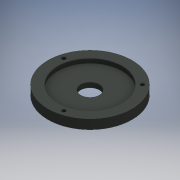
# Autodesk Inventor part: fix_plate
Saved by Autodesk Inventor 2018 (Build 220112000, 112)
## iProperties
Created: 2019-01-08
Part Number: fix_plate
Material: 一般
Document SubType Name: Modeling
Designer: lowyu
Density: 1 g/cm^3
Appearance: 既定
Author: lowyu
Autodesk Inventor part; units mm, degrees
ref_plane "YZ Plane" through (0, 0, 0) normal (1, 0, 0) x (0, 1, 0)
ref_plane "XZ Plane" through (0, 0, 0) normal (0, 1, 0) x (-1, 0, 0)
ref_plane "XY Plane" through (0, 0, 0) normal (0, 0, 1) x (1, 0, 0)
sketch "スケッチ1" plane through (0, 0, 0) normal (0, 0, 1) x (1, 0, 0)
  circle A0 centre (0, 0) radius 46.9412
  dimension "d3" = 93.8824
  constraints: 1 centre point
  measures "d3" diameter of A0
extrude "押し出し1" add sketch "スケッチ1" along normal blind 10.5
sketch "スケッチ2" plane through (0, 0, 10.5) normal (0, 0, 1) x (1, 0, 0)
  circle A0 centre (0, 0) radius 46.9412
  arc A1 (-5.0225, 35.5945) -> (35.5945, -5.0225) centre (0, 0) ccw
  arc A2 (35.7361, 3.8892) -> (3.8892, 35.7361) centre (0, 0) ccw
  circle A3 centre (29.2617, 29.2617) radius 2.1
  circle A4 centre (-39.9723, 10.7105) radius 2.1
  circle A5 centre (10.7105, -39.9723) radius 2.1
  circle A6 centre (0, 0) radius 35.9471
  dimension "d4" = 4.2
  constraints: 6 centre point, 4 point on circle, 1 coincident, 3 other
  measures "d4" diameter of A3
extrude "押し出し2" cut sketch "スケッチ2" against normal blind 5 contours A6 A2 A1
sketch "スケッチ3" plane through (0, 0, 10.5) normal (0, 0, 1) x (1, 0, 0)
  circle A0 centre (0, 0) radius 46.9412
  arc A1 (-5.0225, 35.5945) -> (35.5945, -5.0225) centre (0, 0) ccw
  arc A2 (35.7361, 3.8892) -> (3.8892, 35.7361) centre (0, 0) ccw
  circle A3 centre (29.2617, 29.2617) radius 2.1
  circle A4 centre (-39.9723, 10.7105) radius 2.1
  circle A5 centre (10.7105, -39.9723) radius 2.1
  circle A6 centre (0, 0) radius 35.9471
  dimension "d7" = 4.2
  constraints: 6 centre point, 4 point on circle, 1 coincident, 3 other
  measures "d7" diameter of A3
extrude "押し出し3" cut sketch "スケッチ3" against normal blind 10.5 contours A3 | A4 | A5
sketch "スケッチ4" plane through (0, 0, 5.5) normal (0, 0, 1) x (1, 0, 0)
  circle A0 centre (0, 0) radius 10.5
  circle A1 centre (0, 0) radius 10.5
  constraints: 2 centre point
extrude "押し出し4" cut sketch "スケッチ4" against normal blind 10.5
